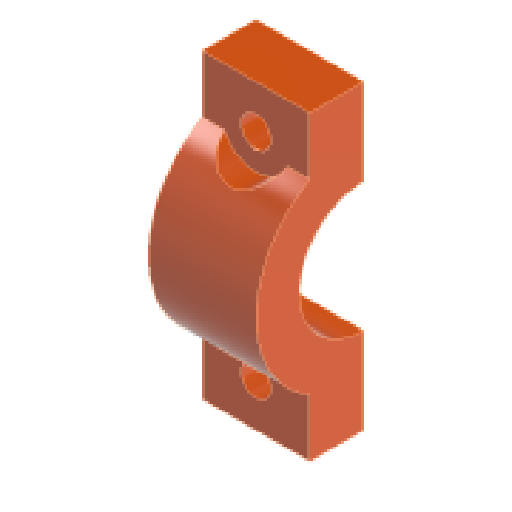
# Autodesk Inventor part: Z Axis Top Brace Clamp
Saved by Autodesk Inventor 2023.2 (Build 272271000, 271)
## iProperties
Created: 2023-02-04
Part Number: Z Axis Top Brace Clamp
Material: ABS Plastic
Document SubType Name: Modeling
Designer: remop
Density: 1.06 g/cm^3
Appearance: Smooth - Light Orange
Author: remop
Autodesk Inventor part; units mm, degrees
ref_plane "YZ Plane" through (0, 0, 0) normal (1, 0, 0) x (0, 1, 0)
ref_plane "XZ Plane" through (0, 0, 0) normal (0, 1, 0) x (-1, 0, 0)
ref_plane "XY Plane" through (0, 0, 0) normal (0, 0, 1) x (1, 0, 0)
sketch "Sketch1" plane through (0, 0, 0) normal (0, 0, 1) x (1, 0, 0)
  circle A0 centre (-5, -16) radius 1.4 projected
  line L0 (0, -20) -> (0, -12) projected
  line L1 (0, -12) -> (-10, -12) projected
  line L2 (-10, -20) -> (-10, -12) projected
  line L3 (0, -20) -> (-10, -20) projected
  circle A1 centre (-5, 4) radius 1.4 projected
  line L4 (0, 0) -> (0, 8) projected
  line L5 (0, 8) -> (-10, 8) projected
  line L6 (-10, 0) -> (-10, 8) projected
  line L7 (0, 0) -> (-10, 0) projected
extrude "Extrusion1" add sketch "Sketch1" along normal blind 5
sketch "Sketch2" plane through (-10, -20, 0) normal (-1, 0, 0) x (0, 0, 1)
  line L0 (0, 8) -> (0, 0) projected
  line L1 (0, 0) -> (5, 0) projected
  line L2 (5, 8) -> (5, 0) projected
  line L3 (0, 8) -> (5, 8) projected
  line L4 (0, 28) -> (0, 20) projected
  line L5 (0, 20) -> (5, 20) projected
  line L6 (5, 28) -> (5, 20) projected
  line L7 (0, 28) -> (5, 28) projected
  circle A0 centre (0, 14) radius 6 projected
  circle A1 centre (0, 14) radius 10
  point P0 (5, 22.6603)
  point P1 (5, 5.3397)
  dimension "d2" = 4
  constraints: 1 centre point, 1 coincident
  measures "d2" radial gap between concentric circles of A1 A0
extrude "Extrusion2" add sketch "Sketch2" against normal up to surface (10 mm away) contours A0 L5 L6 A1 L2 L3
sketch "Sketch3" plane through (0, 0, 5) normal (0, 0, 1) x (1, 0, 0)
  line L0 (-5.4063, -14.6603) -> (-10, -14.6603) projected
  line L1 (-10, -14.6603) -> (-10, -20) projected
  line L2 (-10, -20) -> (0, -20) projected
  line L3 (0, -20) -> (0, -14.6603) projected
  line L4 (0, -14.6603) -> (-4.5937, -14.6603) projected
  arc A0 (-5.4063, -14.6603) -> (-4.5937, -14.6603) centre (-5, -16) ccw projected
  line L5 (-10, 2.6603) -> (-5.4063, 2.6603) projected
  arc A1 (-4.5937, 2.6603) -> (-5.4063, 2.6603) centre (-5, 4) ccw projected
  line L6 (-4.5937, 2.6603) -> (0, 2.6603) projected
  line L7 (0, 2.6603) -> (0, 8) projected
  line L8 (0, 8) -> (-10, 8) projected
  line L9 (-10, 8) -> (-10, 2.6603) projected
  circle A2 centre (-5, -16) radius 3.25
  circle A3 centre (-5, 4) radius 1.4 projected
  circle A4 centre (-5, 4) radius 3.25
  point P0 (0, 0)
  point P1 (-7.961, 2.6603)
  point P2 (-2.039, 2.6603)
  point P3 (-2.039, -14.6603)
  point P4 (-7.961, -14.6603)
  dimension "d5" = 6.5
  constraints: 2 centre point, 2 coincident, 1 equal radius
  measures "d5" diameter of A2
extrude "Extrusion3" cut sketch "Sketch3" along normal blind 10 contours L0 A2 L4 A0 | L5 A3 L6 A4 picked at (-4.8549, -16.4084)
body "Solid1"
